Autodesk Inventor part; units mm, degrees
(part 2 of 3)
  line L717 (-49.225, -33.8) -> (-47.975, -33.8)
  line L718 (-47.975, -33.8) -> (-47.975, -32.7)
  line L719 (-47.975, -32.7) -> (-49.225, -32.7)
  arc A261 (-49.425, -32.5) -> (-49.225, -32.7) centre (-49.225, -32.5) ccw
  line L720 (-49.425, -32.5) -> (-49.425, -31.35)
  line L721 (-49.425, -31.35) -> (-50.325, -31.35)
  line L722 (-50.325, -31.35) -> (-50.325, -32.5)
  arc A262 (-50.525, -32.7) -> (-50.325, -32.5) centre (-50.525, -32.5) ccw
  line L723 (-50.525, -32.7) -> (-51.775, -32.7)
  line L724 (-51.775, -32.7) -> (-51.775, -33.8)
  line L725 (-51.775, -33.8) -> (-50.525, -33.8)
  arc A263 (-50.325, -34) -> (-50.525, -33.8) centre (-50.525, -34) ccw
  line L726 (-36.075, -53) -> (-36.075, -54.15)
  line L727 (-36.075, -54.15) -> (-35.175, -54.15)
  line L728 (-35.175, -54.15) -> (-35.175, -53)
  arc A264 (-34.975, -52.8) -> (-35.175, -53) centre (-34.975, -53) ccw
  line L729 (-34.975, -52.8) -> (-33.725, -52.8)
  line L730 (-33.725, -52.8) -> (-33.725, -51.7)
  line L731 (-33.725, -51.7) -> (-34.975, -51.7)
  arc A265 (-35.175, -51.5) -> (-34.975, -51.7) centre (-34.975, -51.5) ccw
  line L732 (-35.175, -51.5) -> (-35.175, -50.35)
  line L733 (-35.175, -50.35) -> (-36.075, -50.35)
  line L734 (-36.075, -50.35) -> (-36.075, -51.5)
  arc A266 (-36.275, -51.7) -> (-36.075, -51.5) centre (-36.275, -51.5) ccw
  line L735 (-36.275, -51.7) -> (-37.525, -51.7)
  line L736 (-37.525, -51.7) -> (-37.525, -52.8)
  line L737 (-37.525, -52.8) -> (-36.275, -52.8)
  arc A267 (-36.075, -53) -> (-36.275, -52.8) centre (-36.275, -53) ccw
  line L738 (-12.325, -53) -> (-12.325, -54.15)
  line L739 (-12.325, -54.15) -> (-11.425, -54.15)
  line L740 (-11.425, -54.15) -> (-11.425, -53)
  arc A268 (-11.225, -52.8) -> (-11.425, -53) centre (-11.225, -53) ccw
  line L741 (-11.225, -52.8) -> (-9.975, -52.8)
  line L742 (-9.975, -52.8) -> (-9.975, -51.7)
  line L743 (-9.975, -51.7) -> (-11.225, -51.7)
  arc A269 (-11.425, -51.5) -> (-11.225, -51.7) centre (-11.225, -51.5) ccw
  line L744 (-11.425, -51.5) -> (-11.425, -50.35)
  line L745 (-11.425, -50.35) -> (-12.325, -50.35)
  line L746 (-12.325, -50.35) -> (-12.325, -51.5)
  arc A270 (-12.525, -51.7) -> (-12.325, -51.5) centre (-12.525, -51.5) ccw
  line L747 (-12.525, -51.7) -> (-13.775, -51.7)
  line L748 (-13.775, -51.7) -> (-13.775, -52.8)
  line L749 (-13.775, -52.8) -> (-12.525, -52.8)
  arc A271 (-12.325, -53) -> (-12.525, -52.8) centre (-12.525, -53) ccw
  line L750 (-19.45, -34) -> (-19.45, -35.15)
  line L751 (-19.45, -35.15) -> (-18.55, -35.15)
  line L752 (-18.55, -35.15) -> (-18.55, -34)
  arc A272 (-18.35, -33.8) -> (-18.55, -34) centre (-18.35, -34) ccw
  line L753 (-18.35, -33.8) -> (-17.1, -33.8)
  line L754 (-17.1, -33.8) -> (-17.1, -32.7)
  line L755 (-17.1, -32.7) -> (-18.35, -32.7)
  arc A273 (-18.55, -32.5) -> (-18.35, -32.7) centre (-18.35, -32.5) ccw
  line L756 (-18.55, -32.5) -> (-18.55, -31.35)
  line L757 (-18.55, -31.35) -> (-19.45, -31.35)
  line L758 (-19.45, -31.35) -> (-19.45, -32.5)
  arc A274 (-19.65, -32.7) -> (-19.45, -32.5) centre (-19.65, -32.5) ccw
  line L759 (-19.65, -32.7) -> (-20.9, -32.7)
  line L760 (-20.9, -32.7) -> (-20.9, -33.8)
  line L761 (-20.9, -33.8) -> (-19.65, -33.8)
  arc A275 (-19.45, -34) -> (-19.65, -33.8) centre (-19.65, -34) ccw
  line L762 (-28.95, -15) -> (-28.95, -16.15)
  line L763 (-28.95, -16.15) -> (-28.05, -16.15)
  line L764 (-28.05, -16.15) -> (-28.05, -15)
  arc A276 (-27.85, -14.8) -> (-28.05, -15) centre (-27.85, -15) ccw
  line L765 (-27.85, -14.8) -> (-26.6, -14.8)
  line L766 (-26.6, -14.8) -> (-26.6, -13.7)
  line L767 (-26.6, -13.7) -> (-27.85, -13.7)
  arc A277 (-28.05, -13.5) -> (-27.85, -13.7) centre (-27.85, -13.5) ccw
  line L768 (-28.05, -13.5) -> (-28.05, -12.35)
  line L769 (-28.05, -12.35) -> (-28.95, -12.35)
  line L770 (-28.95, -12.35) -> (-28.95, -13.5)
  arc A278 (-29.15, -13.7) -> (-28.95, -13.5) centre (-29.15, -13.5) ccw
  line L771 (-29.15, -13.7) -> (-30.4, -13.7)
  line L772 (-30.4, -13.7) -> (-30.4, -14.8)
  line L773 (-30.4, -14.8) -> (-29.15, -14.8)
  arc A279 (-28.95, -15) -> (-29.15, -14.8) centre (-29.15, -15) ccw
  line L774 (-33.7, 4) -> (-33.7, 2.85)
  line L775 (-33.7, 2.85) -> (-32.8, 2.85)
  line L776 (-32.8, 2.85) -> (-32.8, 4)
  arc A280 (-32.6, 4.2) -> (-32.8, 4) centre (-32.6, 4) ccw
  line L777 (-32.6, 4.2) -> (-31.35, 4.2)
  line L778 (-31.35, 4.2) -> (-31.35, 5.3)
  line L779 (-31.35, 5.3) -> (-32.6, 5.3)
  arc A281 (-32.8, 5.5) -> (-32.6, 5.3) centre (-32.6, 5.5) ccw
  line L780 (-32.8, 5.5) -> (-32.8, 6.65)
  line L781 (-32.8, 6.65) -> (-33.7, 6.65)
  line L782 (-33.7, 6.65) -> (-33.7, 5.5)
  arc A282 (-33.9, 5.3) -> (-33.7, 5.5) centre (-33.9, 5.5) ccw
  line L783 (-33.9, 5.3) -> (-35.15, 5.3)
  line L784 (-35.15, 5.3) -> (-35.15, 4.2)
  line L785 (-35.15, 4.2) -> (-33.9, 4.2)
  arc A283 (-33.7, 4) -> (-33.9, 4.2) centre (-33.9, 4) ccw
  line L786 (-14.7, 4) -> (-14.7, 2.85)
  line L787 (-14.7, 2.85) -> (-13.8, 2.85)
  line L788 (-13.8, 2.85) -> (-13.8, 4)
  arc A284 (-13.6, 4.2) -> (-13.8, 4) centre (-13.6, 4) ccw
  line L789 (-13.6, 4.2) -> (-12.35, 4.2)
  line L790 (-12.35, 4.2) -> (-12.35, 5.3)
  line L791 (-12.35, 5.3) -> (-13.6, 5.3)
  arc A285 (-13.8, 5.5) -> (-13.6, 5.3) centre (-13.6, 5.5) ccw
  line L792 (-13.8, 5.5) -> (-13.8, 6.65)
  line L793 (-13.8, 6.65) -> (-14.7, 6.65)
  line L794 (-14.7, 6.65) -> (-14.7, 5.5)
  arc A286 (-14.9, 5.3) -> (-14.7, 5.5) centre (-14.9, 5.5) ccw
  line L795 (-14.9, 5.3) -> (-16.15, 5.3)
  line L796 (-16.15, 5.3) -> (-16.15, 4.2)
  line L797 (-16.15, 4.2) -> (-14.9, 4.2)
  arc A287 (-14.7, 4) -> (-14.9, 4.2) centre (-14.9, 4) ccw
  line L798 (-9.95, -15) -> (-9.95, -16.15)
  line L799 (-9.95, -16.15) -> (-9.05, -16.15)
  line L800 (-9.05, -16.15) -> (-9.05, -15)
  arc A288 (-8.85, -14.8) -> (-9.05, -15) centre (-8.85, -15) ccw
  line L801 (-8.85, -14.8) -> (-7.6, -14.8)
  line L802 (-7.6, -14.8) -> (-7.6, -13.7)
  line L803 (-7.6, -13.7) -> (-8.85, -13.7)
  arc A289 (-9.05, -13.5) -> (-8.85, -13.7) centre (-8.85, -13.5) ccw
  line L804 (-9.05, -13.5) -> (-9.05, -12.35)
  line L805 (-9.05, -12.35) -> (-9.95, -12.35)
  line L806 (-9.95, -12.35) -> (-9.95, -13.5)
  arc A290 (-10.15, -13.7) -> (-9.95, -13.5) centre (-10.15, -13.5) ccw
  line L807 (-10.15, -13.7) -> (-11.4, -13.7)
  line L808 (-11.4, -13.7) -> (-11.4, -14.8)
  line L809 (-11.4, -14.8) -> (-10.15, -14.8)
  arc A291 (-9.95, -15) -> (-10.15, -14.8) centre (-10.15, -15) ccw
  line L810 (9.05, -15) -> (9.05, -16.15)
  line L811 (9.05, -16.15) -> (9.95, -16.15)
  line L812 (9.95, -16.15) -> (9.95, -15)
  arc A292 (10.15, -14.8) -> (9.95, -15) centre (10.15, -15) ccw
  line L813 (10.15, -14.8) -> (11.4, -14.8)
  line L814 (11.4, -14.8) -> (11.4, -13.7)
  line L815 (11.4, -13.7) -> (10.15, -13.7)
  arc A293 (9.95, -13.5) -> (10.15, -13.7) centre (10.15, -13.5) ccw
  line L816 (9.95, -13.5) -> (9.95, -12.35)
  line L817 (9.95, -12.35) -> (9.05, -12.35)
  line L818 (9.05, -12.35) -> (9.05, -13.5)
  arc A294 (8.85, -13.7) -> (9.05, -13.5) centre (8.85, -13.5) ccw
  line L819 (8.85, -13.7) -> (7.6, -13.7)
  line L820 (7.6, -13.7) -> (7.6, -14.8)
  line L821 (7.6, -14.8) -> (8.85, -14.8)
  arc A295 (9.05, -15) -> (8.85, -14.8) centre (8.85, -15) ccw
  line L822 (4.3, 4) -> (4.3, 2.85)
  line L823 (4.3, 2.85) -> (5.2, 2.85)
  line L824 (5.2, 2.85) -> (5.2, 4)
  arc A296 (5.4, 4.2) -> (5.2, 4) centre (5.4, 4) ccw
  line L825 (5.4, 4.2) -> (6.65, 4.2)
  line L826 (6.65, 4.2) -> (6.65, 5.3)
  line L827 (6.65, 5.3) -> (5.4, 5.3)
  arc A297 (5.2, 5.5) -> (5.4, 5.3) centre (5.4, 5.5) ccw
  line L828 (5.2, 5.5) -> (5.2, 6.65)
  line L829 (5.2, 6.65) -> (4.3, 6.65)
  line L830 (4.3, 6.65) -> (4.3, 5.5)
  arc A298 (4.1, 5.3) -> (4.3, 5.5) centre (4.1, 5.5) ccw
  line L831 (4.1, 5.3) -> (2.85, 5.3)
  line L832 (2.85, 5.3) -> (2.85, 4.2)
  line L833 (2.85, 4.2) -> (4.1, 4.2)
  arc A299 (4.3, 4) -> (4.1, 4.2) centre (4.1, 4) ccw
  line L834 (-0.45, -34) -> (-0.45, -35.15)
  line L835 (-0.45, -35.15) -> (0.45, -35.15)
  line L836 (0.45, -35.15) -> (0.45, -34)
  arc A300 (0.65, -33.8) -> (0.45, -34) centre (0.65, -34) ccw
  line L837 (0.65, -33.8) -> (1.9, -33.8)
  line L838 (1.9, -33.8) -> (1.9, -32.7)
  line L839 (1.9, -32.7) -> (0.65, -32.7)
  arc A301 (0.45, -32.5) -> (0.65, -32.7) centre (0.65, -32.5) ccw
  line L840 (0.45, -32.5) -> (0.45, -31.35)
  line L841 (0.45, -31.35) -> (-0.45, -31.35)
  line L842 (-0.45, -31.35) -> (-0.45, -32.5)
  arc A302 (-0.65, -32.7) -> (-0.45, -32.5) centre (-0.65, -32.5) ccw
  line L843 (-0.65, -32.7) -> (-1.9, -32.7)
  line L844 (-1.9, -32.7) -> (-1.9, -33.8)
  line L845 (-1.9, -33.8) -> (-0.65, -33.8)
  arc A303 (-0.45, -34) -> (-0.65, -33.8) centre (-0.65, -34) ccw
  line L846 (18.55, -34) -> (18.55, -35.15)
  line L847 (18.55, -35.15) -> (19.45, -35.15)
  line L848 (19.45, -35.15) -> (19.45, -34)
  arc A304 (19.65, -33.8) -> (19.45, -34) centre (19.65, -34) ccw
  line L849 (19.65, -33.8) -> (20.9, -33.8)
  line L850 (20.9, -33.8) -> (20.9, -32.7)
  line L851 (20.9, -32.7) -> (19.65, -32.7)
  arc A305 (19.45, -32.5) -> (19.65, -32.7) centre (19.65, -32.5) ccw
  line L852 (19.45, -32.5) -> (19.45, -31.35)
  line L853 (19.45, -31.35) -> (18.55, -31.35)
  line L854 (18.55, -31.35) -> (18.55, -32.5)
  arc A306 (18.35, -32.7) -> (18.55, -32.5) centre (18.35, -32.5) ccw
  line L855 (18.35, -32.7) -> (17.1, -32.7)
  line L856 (17.1, -32.7) -> (17.1, -33.8)
  line L857 (17.1, -33.8) -> (18.35, -33.8)
  arc A307 (18.55, -34) -> (18.35, -33.8) centre (18.35, -34) ccw
  line L858 (28.05, -15) -> (28.05, -16.15)
  line L859 (28.05, -16.15) -> (28.95, -16.15)
  line L860 (28.95, -16.15) -> (28.95, -15)
  arc A308 (29.15, -14.8) -> (28.95, -15) centre (29.15, -15) ccw
  line L861 (29.15, -14.8) -> (30.4, -14.8)
  line L862 (30.4, -14.8) -> (30.4, -13.7)
  line L863 (30.4, -13.7) -> (29.15, -13.7)
  arc A309 (28.95, -13.5) -> (29.15, -13.7) centre (29.15, -13.5) ccw
  line L864 (28.95, -13.5) -> (28.95, -12.35)
  line L865 (28.95, -12.35) -> (28.05, -12.35)
  line L866 (28.05, -12.35) -> (28.05, -13.5)
  arc A310 (27.85, -13.7) -> (28.05, -13.5) centre (27.85, -13.5) ccw
  line L867 (27.85, -13.7) -> (26.6, -13.7)
  line L868 (26.6, -13.7) -> (26.6, -14.8)
  line L869 (26.6, -14.8) -> (27.85, -14.8)
  arc A311 (28.05, -15) -> (27.85, -14.8) centre (27.85, -15) ccw
  line L870 (23.3, 4) -> (23.3, 2.85)
  line L871 (23.3, 2.85) -> (24.2, 2.85)
  line L872 (24.2, 2.85) -> (24.2, 4)
  arc A312 (24.4, 4.2) -> (24.2, 4) centre (24.4, 4) ccw
  line L873 (24.4, 4.2) -> (25.65, 4.2)
  line L874 (25.65, 4.2) -> (25.65, 5.3)
  line L875 (25.65, 5.3) -> (24.4, 5.3)
  arc A313 (24.2, 5.5) -> (24.4, 5.3) centre (24.4, 5.5) ccw
  line L876 (24.2, 5.5) -> (24.2, 6.65)
  line L877 (24.2, 6.65) -> (23.3, 6.65)
  line L878 (23.3, 6.65) -> (23.3, 5.5)
  arc A314 (23.1, 5.3) -> (23.3, 5.5) centre (23.1, 5.5) ccw
  line L879 (23.1, 5.3) -> (21.85, 5.3)
  line L880 (21.85, 5.3) -> (21.85, 4.2)
  line L881 (21.85, 4.2) -> (23.1, 4.2)
  arc A315 (23.3, 4) -> (23.1, 4.2) centre (23.1, 4) ccw
  line L882 (37.55, -34) -> (37.55, -35.15)
  line L883 (37.55, -35.15) -> (38.45, -35.15)
  line L884 (38.45, -35.15) -> (38.45, -34)
  arc A316 (38.65, -33.8) -> (38.45, -34) centre (38.65, -34) ccw
  line L885 (38.65, -33.8) -> (39.9, -33.8)
  line L886 (39.9, -33.8) -> (39.9, -32.7)
  line L887 (39.9, -32.7) -> (38.65, -32.7)
  arc A317 (38.45, -32.5) -> (38.65, -32.7) centre (38.65, -32.5) ccw
  line L888 (38.45, -32.5) -> (38.45, -31.35)
  line L889 (38.45, -31.35) -> (37.55, -31.35)
  line L890 (37.55, -31.35) -> (37.55, -32.5)
  arc A318 (37.35, -32.7) -> (37.55, -32.5) centre (37.35, -32.5) ccw
  line L891 (37.35, -32.7) -> (36.1, -32.7)
  line L892 (36.1, -32.7) -> (36.1, -33.8)
  line L893 (36.1, -33.8) -> (37.35, -33.8)
  arc A319 (37.55, -34) -> (37.35, -33.8) centre (37.35, -34) ccw
  line L894 (47.05, -15) -> (47.05, -16.15)
  line L895 (47.05, -16.15) -> (47.95, -16.15)
  line L896 (47.95, -16.15) -> (47.95, -15)
  arc A320 (48.15, -14.8) -> (47.95, -15) centre (48.15, -15) ccw
  line L897 (48.15, -14.8) -> (49.4, -14.8)
  line L898 (49.4, -14.8) -> (49.4, -13.7)
  line L899 (49.4, -13.7) -> (48.15, -13.7)
  arc A321 (47.95, -13.5) -> (48.15, -13.7) centre (48.15, -13.5) ccw
  line L900 (47.95, -13.5) -> (47.95, -12.35)
  line L901 (47.95, -12.35) -> (47.05, -12.35)
  line L902 (47.05, -12.35) -> (47.05, -13.5)
  arc A322 (46.85, -13.7) -> (47.05, -13.5) centre (46.85, -13.5) ccw
  line L903 (46.85, -13.7) -> (45.6, -13.7)
  line L904 (45.6, -13.7) -> (45.6, -14.8)
  line L905 (45.6, -14.8) -> (46.85, -14.8)
  arc A323 (47.05, -15) -> (46.85, -14.8) centre (46.85, -15) ccw
  line L906 (42.3, 4) -> (42.3, 2.85)
  line L907 (42.3, 2.85) -> (43.2, 2.85)
  line L908 (43.2, 2.85) -> (43.2, 4)
  arc A324 (43.4, 4.2) -> (43.2, 4) centre (43.4, 4) ccw
  line L909 (43.4, 4.2) -> (44.65, 4.2)
  line L910 (44.65, 4.2) -> (44.65, 5.3)
  line L911 (44.65, 5.3) -> (43.4, 5.3)
  arc A325 (43.2, 5.5) -> (43.4, 5.3) centre (43.4, 5.5) ccw
  line L912 (43.2, 5.5) -> (43.2, 6.65)
  line L913 (43.2, 6.65) -> (42.3, 6.65)
  line L914 (42.3, 6.65) -> (42.3, 5.5)
  arc A326 (42.1, 5.3) -> (42.3, 5.5) centre (42.1, 5.5) ccw
  line L915 (42.1, 5.3) -> (40.85, 5.3)
  line L916 (40.85, 5.3) -> (40.85, 4.2)
  line L917 (40.85, 4.2) -> (42.1, 4.2)
  arc A327 (42.3, 4) -> (42.1, 4.2) centre (42.1, 4) ccw
  line L918 (61.3, 4) -> (61.3, 2.85)
  line L919 (61.3, 2.85) -> (62.2, 2.85)
  line L920 (62.2, 2.85) -> (62.2, 4)
  arc A328 (62.4, 4.2) -> (62.2, 4) centre (62.4, 4) ccw
  line L921 (62.4, 4.2) -> (63.65, 4.2)
  line L922 (63.65, 4.2) -> (63.65, 5.3)
  line L923 (63.65, 5.3) -> (62.4, 5.3)
  arc A329 (62.2, 5.5) -> (62.4, 5.3) centre (62.4, 5.5) ccw
  line L924 (62.2, 5.5) -> (62.2, 6.65)
  line L925 (62.2, 6.65) -> (61.3, 6.65)
  line L926 (61.3, 6.65) -> (61.3, 5.5)
  arc A330 (61.1, 5.3) -> (61.3, 5.5) centre (61.1, 5.5) ccw
  line L927 (61.1, 5.3) -> (59.85, 5.3)
  line L928 (59.85, 5.3) -> (59.85, 4.2)
  line L929 (59.85, 4.2) -> (61.1, 4.2)
  arc A331 (61.3, 4) -> (61.1, 4.2) centre (61.1, 4) ccw
  line L930 (80.3, 4) -> (80.3, 2.85)
  line L931 (80.3, 2.85) -> (81.2, 2.85)
  line L932 (81.2, 2.85) -> (81.2, 4)
  arc A332 (81.4, 4.2) -> (81.2, 4) centre (81.4, 4) ccw
  line L933 (81.4, 4.2) -> (82.65, 4.2)
  line L934 (82.65, 4.2) -> (82.65, 5.3)
  line L935 (82.65, 5.3) -> (81.4, 5.3)
  arc A333 (81.2, 5.5) -> (81.4, 5.3) centre (81.4, 5.5) ccw
  line L936 (81.2, 5.5) -> (81.2, 6.65)
  line L937 (81.2, 6.65) -> (80.3, 6.65)
  line L938 (80.3, 6.65) -> (80.3, 5.5)
  arc A334 (80.1, 5.3) -> (80.3, 5.5) centre (80.1, 5.5) ccw
  line L939 (80.1, 5.3) -> (78.85, 5.3)
  line L940 (78.85, 5.3) -> (78.85, 4.2)
  line L941 (78.85, 4.2) -> (80.1, 4.2)
  arc A335 (80.3, 4) -> (80.1, 4.2) centre (80.1, 4) ccw
  line L942 (85.05, -15) -> (85.05, -16.15)
  line L943 (85.05, -16.15) -> (85.95, -16.15)
  line L944 (85.95, -16.15) -> (85.95, -15)
  arc A336 (86.15, -14.8) -> (85.95, -15) centre (86.15, -15) ccw
  line L945 (86.15, -14.8) -> (87.4, -14.8)
  line L946 (87.4, -14.8) -> (87.4, -13.7)
  line L947 (87.4, -13.7) -> (86.15, -13.7)
  arc A337 (85.95, -13.5) -> (86.15, -13.7) centre (86.15, -13.5) ccw
  line L948 (85.95, -13.5) -> (85.95, -12.35)
  line L949 (85.95, -12.35) -> (85.05, -12.35)
  line L950 (85.05, -12.35) -> (85.05, -13.5)
  arc A338 (84.85, -13.7) -> (85.05, -13.5) centre (84.85, -13.5) ccw
  line L951 (84.85, -13.7) -> (83.6, -13.7)
  line L952 (83.6, -13.7) -> (83.6, -14.8)
  line L953 (83.6, -14.8) -> (84.85, -14.8)
  arc A339 (85.05, -15) -> (84.85, -14.8) centre (84.85, -15) ccw
  line L954 (66.05, -15) -> (66.05, -16.15)
  line L955 (66.05, -16.15) -> (66.95, -16.15)
  line L956 (66.95, -16.15) -> (66.95, -15)
  arc A340 (67.15, -14.8) -> (66.95, -15) centre (67.15, -15) ccw
  line L957 (67.15, -14.8) -> (68.4, -14.8)
  line L958 (68.4, -14.8) -> (68.4, -13.7)
  line L959 (68.4, -13.7) -> (67.15, -13.7)
  arc A341 (66.95, -13.5) -> (67.15, -13.7) centre (67.15, -13.5) ccw
  line L960 (66.95, -13.5) -> (66.95, -12.35)
  line L961 (66.95, -12.35) -> (66.05, -12.35)
  line L962 (66.05, -12.35) -> (66.05, -13.5)
  arc A342 (65.85, -13.7) -> (66.05, -13.5) centre (65.85, -13.5) ccw
  line L963 (65.85, -13.7) -> (64.6, -13.7)
  line L964 (64.6, -13.7) -> (64.6, -14.8)
  line L965 (64.6, -14.8) -> (65.85, -14.8)
  arc A343 (66.05, -15) -> (65.85, -14.8) centre (65.85, -15) ccw
  line L966 (56.55, -34) -> (56.55, -35.15)
  line L967 (56.55, -35.15) -> (57.45, -35.15)
  line L968 (57.45, -35.15) -> (57.45, -34)
  arc A344 (57.65, -33.8) -> (57.45, -34) centre (57.65, -34) ccw
  line L969 (57.65, -33.8) -> (58.9, -33.8)
  line L970 (58.9, -33.8) -> (58.9, -32.7)
  line L971 (58.9, -32.7) -> (57.65, -32.7)
  arc A345 (57.45, -32.5) -> (57.65, -32.7) centre (57.65, -32.5) ccw
  line L972 (57.45, -32.5) -> (57.45, -31.35)
  line L973 (57.45, -31.35) -> (56.55, -31.35)
  line L974 (56.55, -31.35) -> (56.55, -32.5)
  arc A346 (56.35, -32.7) -> (56.55, -32.5) centre (56.35, -32.5) ccw
  line L975 (56.35, -32.7) -> (55.1, -32.7)
  line L976 (55.1, -32.7) -> (55.1, -33.8)
  line L977 (55.1, -33.8) -> (56.35, -33.8)
  arc A347 (56.55, -34) -> (56.35, -33.8) centre (56.35, -34) ccw
  line L978 (75.55, -34) -> (75.55, -35.15)
  line L979 (75.55, -35.15) -> (76.45, -35.15)
  line L980 (76.45, -35.15) -> (76.45, -34)
  arc A348 (76.65, -33.8) -> (76.45, -34) centre (76.65, -34) ccw
  line L981 (76.65, -33.8) -> (77.9, -33.8)
  line L982 (77.9, -33.8) -> (77.9, -32.7)
  line L983 (77.9, -32.7) -> (76.65, -32.7)
  arc A349 (76.45, -32.5) -> (76.65, -32.7) centre (76.65, -32.5) ccw
  line L984 (76.45, -32.5) -> (76.45, -31.35)
  line L985 (76.45, -31.35) -> (75.55, -31.35)
  line L986 (75.55, -31.35) -> (75.55, -32.5)
  arc A350 (75.35, -32.7) -> (75.55, -32.5) centre (75.35, -32.5) ccw
  line L987 (75.35, -32.7) -> (74.1, -32.7)
  line L988 (74.1, -32.7) -> (74.1, -33.8)
  line L989 (74.1, -33.8) -> (75.35, -33.8)
  arc A351 (75.55, -34) -> (75.35, -33.8) centre (75.35, -34) ccw
  line L990 (94.55, -34) -> (94.55, -35.15)
  line L991 (94.55, -35.15) -> (95.45, -35.15)
  line L992 (95.45, -35.15) -> (95.45, -34)
  arc A352 (95.65, -33.8) -> (95.45, -34) centre (95.65, -34) ccw
  line L993 (95.65, -33.8) -> (96.9, -33.8)
  line L994 (96.9, -33.8) -> (96.9, -32.7)
  line L995 (96.9, -32.7) -> (95.65, -32.7)
  arc A353 (95.45, -32.5) -> (95.65, -32.7) centre (95.65, -32.5) ccw
  line L996 (95.45, -32.5) -> (95.45, -31.35)
  line L997 (95.45, -31.35) -> (94.55, -31.35)
  line L998 (94.55, -31.35) -> (94.55, -32.5)
  arc A354 (94.35, -32.7) -> (94.55, -32.5) centre (94.35, -32.5) ccw
  line L999 (94.35, -32.7) -> (93.1, -32.7)
  line L1000 (93.1, -32.7) -> (93.1, -33.8)
  line L1001 (93.1, -33.8) -> (94.35, -33.8)
  arc A355 (94.55, -34) -> (94.35, -33.8) centre (94.35, -34) ccw
  line L1002 (104.05, -15) -> (104.05, -16.15)
  line L1003 (104.05, -16.15) -> (104.95, -16.15)
  line L1004 (104.95, -16.15) -> (104.95, -15)
  arc A356 (105.15, -14.8) -> (104.95, -15) centre (105.15, -15) ccw
  line L1005 (105.15, -14.8) -> (106.4, -14.8)
  line L1006 (106.4, -14.8) -> (106.4, -13.7)
  line L1007 (106.4, -13.7) -> (105.15, -13.7)
  arc A357 (104.95, -13.5) -> (105.15, -13.7) centre (105.15, -13.5) ccw
  line L1008 (104.95, -13.5) -> (104.95, -12.35)
  line L1009 (104.95, -12.35) -> (104.05, -12.35)
  line L1010 (104.05, -12.35) -> (104.05, -13.5)
  arc A358 (103.85, -13.7) -> (104.05, -13.5) centre (103.85, -13.5) ccw
  line L1011 (103.85, -13.7) -> (102.6, -13.7)
  line L1012 (102.6, -13.7) -> (102.6, -14.8)
  line L1013 (102.6, -14.8) -> (103.85, -14.8)
  arc A359 (104.05, -15) -> (103.85, -14.8) centre (103.85, -15) ccw
  line L1014 (99.3, 4) -> (99.3, 2.85)
  line L1015 (99.3, 2.85) -> (100.2, 2.85)
  line L1016 (100.2, 2.85) -> (100.2, 4)
  arc A360 (100.4, 4.2) -> (100.2, 4) centre (100.4, 4) ccw
  line L1017 (100.4, 4.2) -> (101.65, 4.2)
  line L1018 (101.65, 4.2) -> (101.65, 5.3)
  line L1019 (101.65, 5.3) -> (100.4, 5.3)
  arc A361 (100.2, 5.5) -> (100.4, 5.3) centre (100.4, 5.5) ccw
  line L1020 (100.2, 5.5) -> (100.2, 6.65)
  line L1021 (100.2, 6.65) -> (99.3, 6.65)
  line L1022 (99.3, 6.65) -> (99.3, 5.5)
  arc A362 (99.1, 5.3) -> (99.3, 5.5) centre (99.1, 5.5) ccw
  line L1023 (99.1, 5.3) -> (97.85, 5.3)
  line L1024 (97.85, 5.3) -> (97.85, 4.2)
  line L1025 (97.85, 4.2) -> (99.1, 4.2)
  arc A363 (99.3, 4) -> (99.1, 4.2) centre (99.1, 4) ccw
  line L1026 (118.3, 4) -> (118.3, 2.85)
  line L1027 (118.3, 2.85) -> (119.2, 2.85)
  line L1028 (119.2, 2.85) -> (119.2, 4)
  arc A364 (119.4, 4.2) -> (119.2, 4) centre (119.4, 4) ccw
  line L1029 (119.4, 4.2) -> (120.65, 4.2)
  line L1030 (120.65, 4.2) -> (120.65, 5.3)
  line L1031 (120.65, 5.3) -> (119.4, 5.3)
  arc A365 (119.2, 5.5) -> (119.4, 5.3) centre (119.4, 5.5) ccw
  line L1032 (119.2, 5.5) -> (119.2, 6.65)
  line L1033 (119.2, 6.65) -> (118.3, 6.65)
  line L1034 (118.3, 6.65) -> (118.3, 5.5)
  arc A366 (118.1, 5.3) -> (118.3, 5.5) centre (118.1, 5.5) ccw
  line L1035 (118.1, 5.3) -> (116.85, 5.3)
  line L1036 (116.85, 5.3) -> (116.85, 4.2)
  line L1037 (116.85, 4.2) -> (118.1, 4.2)
  arc A367 (118.3, 4) -> (118.1, 4.2) centre (118.1, 4) ccw
  line L1038 (137.3, 4) -> (137.3, 2.85)
  line L1039 (137.3, 2.85) -> (138.2, 2.85)
  line L1040 (138.2, 2.85) -> (138.2, 4)
  arc A368 (138.4, 4.2) -> (138.2, 4) centre (138.4, 4) ccw
  line L1041 (138.4, 4.2) -> (139.65, 4.2)
  line L1042 (139.65, 4.2) -> (139.65, 5.3)
  line L1043 (139.65, 5.3) -> (138.4, 5.3)
  arc A369 (138.2, 5.5) -> (138.4, 5.3) centre (138.4, 5.5) ccw
  line L1044 (138.2, 5.5) -> (138.2, 6.65)
  line L1045 (138.2, 6.65) -> (137.3, 6.65)
  line L1046 (137.3, 6.65) -> (137.3, 5.5)
  arc A370 (137.1, 5.3) -> (137.3, 5.5) centre (137.1, 5.5) ccw
  line L1047 (137.1, 5.3) -> (135.85, 5.3)
  line L1048 (135.85, 5.3) -> (135.85, 4.2)
  line L1049 (135.85, 4.2) -> (137.1, 4.2)
  arc A371 (137.3, 4) -> (137.1, 4.2) centre (137.1, 4) ccw
  line L1050 (123.05, -15) -> (123.05, -16.15)
  line L1051 (123.05, -16.15) -> (123.95, -16.15)
  line L1052 (123.95, -16.15) -> (123.95, -15)
  arc A372 (124.15, -14.8) -> (123.95, -15) centre (124.15, -15) ccw
  line L1053 (124.15, -14.8) -> (125.4, -14.8)
  line L1054 (125.4, -14.8) -> (125.4, -13.7)
  line L1055 (125.4, -13.7) -> (124.15, -13.7)
  arc A373 (123.95, -13.5) -> (124.15, -13.7) centre (124.15, -13.5) ccw
  line L1056 (123.95, -13.5) -> (123.95, -12.35)
  line L1057 (123.95, -12.35) -> (123.05, -12.35)
  line L1058 (123.05, -12.35) -> (123.05, -13.5)
  arc A374 (122.85, -13.7) -> (123.05, -13.5) centre (122.85, -13.5) ccw
  line L1059 (122.85, -13.7) -> (121.6, -13.7)
  line L1060 (121.6, -13.7) -> (121.6, -14.8)
  line L1061 (121.6, -14.8) -> (122.85, -14.8)
  arc A375 (123.05, -15) -> (122.85, -14.8) centre (122.85, -15) ccw
  line L1062 (142.05, -15) -> (142.05, -16.15)
  line L1063 (142.05, -16.15) -> (142.95, -16.15)
  line L1064 (142.95, -16.15) -> (142.95, -15)
  arc A376 (143.15, -14.8) -> (142.95, -15) centre (143.15, -15) ccw
  line L1065 (143.15, -14.8) -> (144.4, -14.8)
  line L1066 (144.4, -14.8) -> (144.4, -13.7)
  line L1067 (144.4, -13.7) -> (143.15, -13.7)
  arc A377 (142.95, -13.5) -> (143.15, -13.7) centre (143.15, -13.5) ccw
  line L1068 (142.95, -13.5) -> (142.95, -12.35)
  line L1069 (142.95, -12.35) -> (142.05, -12.35)
  line L1070 (142.05, -12.35) -> (142.05, -13.5)
  arc A378 (141.85, -13.7) -> (142.05, -13.5) centre (141.85, -13.5) ccw
  line L1071 (141.85, -13.7) -> (140.6, -13.7)
  line L1072 (140.6, -13.7) -> (140.6, -14.8)
  line L1073 (140.6, -14.8) -> (141.85, -14.8)
  arc A379 (142.05, -15) -> (141.85, -14.8) centre (141.85, -15) ccw
  line L1074 (156.3, 4) -> (156.3, 2.85)
  line L1075 (156.3, 2.85) -> (157.2, 2.85)
  line L1076 (157.2, 2.85) -> (157.2, 4)
  arc A380 (157.4, 4.2) -> (157.2, 4) centre (157.4, 4) ccw
  line L1077 (157.4, 4.2) -> (158.65, 4.2)
  line L1078 (158.65, 4.2) -> (158.65, 5.3)
  line L1079 (158.65, 5.3) -> (157.4, 5.3)
  arc A381 (157.2, 5.5) -> (157.4, 5.3) centre (157.4, 5.5) ccw
  line L1080 (157.2, 5.5) -> (157.2, 6.65)
  line L1081 (157.2, 6.65) -> (156.3, 6.65)
  line L1082 (156.3, 6.65) -> (156.3, 5.5)
  arc A382 (156.1, 5.3) -> (156.3, 5.5) centre (156.1, 5.5) ccw
  line L1083 (156.1, 5.3) -> (154.85, 5.3)
  line L1084 (154.85, 5.3) -> (154.85, 4.2)
  line L1085 (154.85, 4.2) -> (156.1, 4.2)
  arc A383 (156.3, 4) -> (156.1, 4.2) centre (156.1, 4) ccw
  line L1086 (161.05, -15) -> (161.05, -16.15)
  line L1087 (161.05, -16.15) -> (161.95, -16.15)
  line L1088 (161.95, -16.15) -> (161.95, -15)
  arc A384 (162.15, -14.8) -> (161.95, -15) centre (162.15, -15) ccw
  line L1089 (162.15, -14.8) -> (163.4, -14.8)
  line L1090 (163.4, -14.8) -> (163.4, -13.7)
  line L1091 (163.4, -13.7) -> (162.15, -13.7)
  arc A385 (161.95, -13.5) -> (162.15, -13.7) centre (162.15, -13.5) ccw
  line L1092 (161.95, -13.5) -> (161.95, -12.35)
  line L1093 (161.95, -12.35) -> (161.05, -12.35)
  line L1094 (161.05, -12.35) -> (161.05, -13.5)
  arc A386 (160.85, -13.7) -> (161.05, -13.5) centre (160.85, -13.5) ccw
  line L1095 (160.85, -13.7) -> (159.6, -13.7)
  line L1096 (159.6, -13.7) -> (159.6, -14.8)
  line L1097 (159.6, -14.8) -> (160.85, -14.8)
  arc A387 (161.05, -15) -> (160.85, -14.8) centre (160.85, -15) ccw
  line L1098 (113.55, -34) -> (113.55, -35.15)
  line L1099 (113.55, -35.15) -> (114.45, -35.15)
  line L1100 (114.45, -35.15) -> (114.45, -34)
  arc A388 (114.65, -33.8) -> (114.45, -34) centre (114.65, -34) ccw
  line L1101 (114.65, -33.8) -> (115.9, -33.8)
  line L1102 (115.9, -33.8) -> (115.9, -32.7)
  line L1103 (115.9, -32.7) -> (114.65, -32.7)
  arc A389 (114.45, -32.5) -> (114.65, -32.7) centre (114.65, -32.5) ccw
  line L1104 (114.45, -32.5) -> (114.45, -31.35)
  line L1105 (114.45, -31.35) -> (113.55, -31.35)
  line L1106 (113.55, -31.35) -> (113.55, -32.5)
  arc A390 (113.35, -32.7) -> (113.55, -32.5) centre (113.35, -32.5) ccw
  line L1107 (113.35, -32.7) -> (112.1, -32.7)
  line L1108 (112.1, -32.7) -> (112.1, -33.8)
  line L1109 (112.1, -33.8) -> (113.35, -33.8)
  arc A391 (113.55, -34) -> (113.35, -33.8) centre (113.35, -34) ccw
  line L1110 (132.55, -34) -> (132.55, -35.15)
  line L1111 (132.55, -35.15) -> (133.45, -35.15)
  line L1112 (133.45, -35.15) -> (133.45, -34)
  arc A392 (133.65, -33.8) -> (133.45, -34) centre (133.65, -34) ccw
  line L1113 (133.65, -33.8) -> (134.9, -33.8)
  line L1114 (134.9, -33.8) -> (134.9, -32.7)
  line L1115 (134.9, -32.7) -> (133.65, -32.7)
  arc A393 (133.45, -32.5) -> (133.65, -32.7) centre (133.65, -32.5) ccw
  line L1116 (133.45, -32.5) -> (133.45, -31.35)
  line L1117 (133.45, -31.35) -> (132.55, -31.35)
  line L1118 (132.55, -31.35) -> (132.55, -32.5)
  arc A394 (132.35, -32.7) -> (132.55, -32.5) centre (132.35, -32.5) ccw
  line L1119 (132.35, -32.7) -> (131.1, -32.7)
  line L1120 (131.1, -32.7) -> (131.1, -33.8)
  line L1121 (131.1, -33.8) -> (132.35, -33.8)
  arc A395 (132.55, -34) -> (132.35, -33.8) centre (132.35, -34) ccw
  line L1122 (151.55, -34) -> (151.55, -35.15)
  line L1123 (151.55, -35.15) -> (152.45, -35.15)
  line L1124 (152.45, -35.15) -> (152.45, -34)
  arc A396 (152.65, -33.8) -> (152.45, -34) centre (152.65, -34) ccw
  line L1125 (152.65, -33.8) -> (153.9, -33.8)
  line L1126 (153.9, -33.8) -> (153.9, -32.7)
  line L1127 (153.9, -32.7) -> (152.65, -32.7)
  arc A397 (152.45, -32.5) -> (152.65, -32.7) centre (152.65, -32.5) ccw
  line L1128 (152.45, -32.5) -> (152.45, -31.35)
  line L1129 (152.45, -31.35) -> (151.55, -31.35)
  line L1130 (151.55, -31.35) -> (151.55, -32.5)
  arc A398 (151.35, -32.7) -> (151.55, -32.5) centre (151.35, -32.5) ccw
  line L1131 (151.35, -32.7) -> (150.1, -32.7)
  line L1132 (150.1, -32.7) -> (150.1, -33.8)
  line L1133 (150.1, -33.8) -> (151.35, -33.8)
  arc A399 (151.55, -34) -> (151.35, -33.8) centre (151.35, -34) ccw
  line L1134 (175.3, 4) -> (175.3, 2.85)
  line L1135 (175.3, 2.85) -> (176.2, 2.85)
  line L1136 (176.2, 2.85) -> (176.2, 4)
  arc A400 (176.4, 4.2) -> (176.2, 4) centre (176.4, 4) ccw
  line L1137 (176.4, 4.2) -> (177.65, 4.2)
  line L1138 (177.65, 4.2) -> (177.65, 5.3)
  line L1139 (177.65, 5.3) -> (176.4, 5.3)
  arc A401 (176.2, 5.5) -> (176.4, 5.3) centre (176.4, 5.5) ccw
  line L1140 (176.2, 5.5) -> (176.2, 6.65)
  line L1141 (176.2, 6.65) -> (175.3, 6.65)
  line L1142 (175.3, 6.65) -> (175.3, 5.5)
  arc A402 (175.1, 5.3) -> (175.3, 5.5) centre (175.1, 5.5) ccw
  line L1143 (175.1, 5.3) -> (173.85, 5.3)
  line L1144 (173.85, 5.3) -> (173.85, 4.2)
  line L1145 (173.85, 4.2) -> (175.1, 4.2)
  arc A403 (175.3, 4) -> (175.1, 4.2) centre (175.1, 4) ccw
  line L1146 (199.05, 4) -> (199.05, 2.85)
  line L1147 (199.05, 2.85) -> (199.95, 2.85)
  line L1148 (199.95, 2.85) -> (199.95, 4)
  arc A404 (200.15, 4.2) -> (199.95, 4) centre (200.15, 4) ccw
  line L1149 (200.15, 4.2) -> (201.4, 4.2)
  line L1150 (201.4, 4.2) -> (201.4, 5.3)
  line L1151 (201.4, 5.3) -> (200.15, 5.3)
  arc A405 (199.95, 5.5) -> (200.15, 5.3) centre (200.15, 5.5) ccw
  line L1152 (199.95, 5.5) -> (199.95, 6.65)
  line L1153 (199.95, 6.65) -> (199.05, 6.65)
  line L1154 (199.05, 6.65) -> (199.05, 5.5)
  arc A406 (198.85, 5.3) -> (199.05, 5.5) centre (198.85, 5.5) ccw
  line L1155 (198.85, 5.3) -> (197.6, 5.3)
  line L1156 (197.6, 5.3) -> (197.6, 4.2)
  line L1157 (197.6, 4.2) -> (198.85, 4.2)
  arc A407 (199.05, 4) -> (198.85, 4.2) centre (198.85, 4) ccw
  line L1158 (191.925, -15) -> (191.925, -16.15)
  line L1159 (191.925, -16.15) -> (192.825, -16.15)
  line L1160 (192.825, -16.15) -> (192.825, -15)
  arc A408 (193.025, -14.8) -> (192.825, -15) centre (193.025, -15) ccw
  line L1161 (193.025, -14.8) -> (194.275, -14.8)
  line L1162 (194.275, -14.8) -> (194.275, -13.7)
  line L1163 (194.275, -13.7) -> (193.025, -13.7)
  arc A409 (192.825, -13.5) -> (193.025, -13.7) centre (193.025, -13.5) ccw
  line L1164 (192.825, -13.5) -> (192.825, -12.35)
  line L1165 (192.825, -12.35) -> (191.925, -12.35)
  line L1166 (191.925, -12.35) -> (191.925, -13.5)
  arc A410 (191.725, -13.7) -> (191.925, -13.5) centre (191.725, -13.5) ccw
  line L1167 (191.725, -13.7) -> (190.475, -13.7)
  line L1168 (190.475, -13.7) -> (190.475, -14.8)
  line L1169 (190.475, -14.8) -> (191.725, -14.8)
  arc A411 (191.925, -15) -> (191.725, -14.8) centre (191.725, -15) ccw
  line L1170 (187.175, -34) -> (187.175, -35.15)
  line L1171 (187.175, -35.15) -> (188.075, -35.15)
  line L1172 (188.075, -35.15) -> (188.075, -34)
  arc A412 (188.275, -33.8) -> (188.075, -34) centre (188.275, -34) ccw
  line L1173 (188.275, -33.8) -> (189.525, -33.8)
  line L1174 (189.525, -33.8) -> (189.525, -32.7)
  line L1175 (189.525, -32.7) -> (188.275, -32.7)
  arc A413 (188.075, -32.5) -> (188.275, -32.7) centre (188.275, -32.5) ccw
  line L1176 (188.075, -32.5) -> (188.075, -31.35)
  line L1177 (188.075, -31.35) -> (187.175, -31.35)
  line L1178 (187.175, -31.35) -> (187.175, -32.5)
  arc A414 (186.975, -32.7) -> (187.175, -32.5) centre (186.975, -32.5) ccw
  line L1179 (186.975, -32.7) -> (185.725, -32.7)
  line L1180 (185.725, -32.7) -> (185.725, -33.8)
  line L1181 (185.725, -33.8) -> (186.975, -33.8)
  arc A415 (187.175, -34) -> (186.975, -33.8) centre (186.975, -34) ccw
  line L1182 (201.425, -53) -> (201.425, -54.15)
  line L1183 (201.425, -54.15) -> (202.325, -54.15)
  line L1184 (202.325, -54.15) -> (202.325, -53)
  arc A416 (202.525, -52.8) -> (202.325, -53) centre (202.525, -53) ccw
  line L1185 (202.525, -52.8) -> (203.775, -52.8)
  line L1186 (203.775, -52.8) -> (203.775, -51.7)
  line L1187 (203.775, -51.7) -> (202.525, -51.7)
  arc A417 (202.325, -51.5) -> (202.525, -51.7) centre (202.525, -51.5) ccw
  line L1188 (202.325, -51.5) -> (202.325, -50.35)
  line L1189 (202.325, -50.35) -> (201.425, -50.35)
  line L1190 (201.425, -50.35) -> (201.425, -51.5)
  arc A418 (201.225, -51.7) -> (201.425, -51.5) centre (201.225, -51.5) ccw
  line L1191 (201.225, -51.7) -> (199.975, -51.7)
  line L1192 (199.975, -51.7) -> (199.975, -52.8)
  line L1193 (199.975, -52.8) -> (201.225, -52.8)
  arc A419 (201.425, -53) -> (201.225, -52.8) centre (201.225, -53) ccw
  line L1194 (177.675, -53) -> (177.675, -54.15)
  line L1195 (177.675, -54.15) -> (178.575, -54.15)
  line L1196 (178.575, -54.15) -> (178.575, -53)
  arc A420 (178.775, -52.8) -> (178.575, -53) centre (178.775, -53) ccw
  line L1197 (178.775, -52.8) -> (180.025, -52.8)
  line L1198 (180.025, -52.8) -> (180.025, -51.7)
  line L1199 (180.025, -51.7) -> (178.775, -51.7)
  arc A421 (178.575, -51.5) -> (178.775, -51.7) centre (178.775, -51.5) ccw
  line L1200 (178.575, -51.5) -> (178.575, -50.35)
  line L1201 (178.575, -50.35) -> (177.675, -50.35)
  line L1202 (177.675, -50.35) -> (177.675, -51.5)
  arc A422 (177.475, -51.7) -> (177.675, -51.5) centre (177.475, -51.5) ccw
  line L1203 (177.475, -51.7) -> (176.225, -51.7)
  line L1204 (176.225, -51.7) -> (176.225, -52.8)
  line L1205 (176.225, -52.8) -> (177.475, -52.8)
  arc A423 (177.675, -53) -> (177.475, -52.8) centre (177.475, -53) ccw
  line L1206 (153.925, -53) -> (153.925, -54.15)
  line L1207 (153.925, -54.15) -> (154.825, -54.15)
  line L1208 (154.825, -54.15) -> (154.825, -53)
  arc A424 (155.025, -52.8) -> (154.825, -53) centre (155.025, -53) ccw
  line L1209 (155.025, -52.8) -> (156.275, -52.8)
  line L1210 (156.275, -52.8) -> (156.275, -51.7)
  line L1211 (156.275, -51.7) -> (155.025, -51.7)
  arc A425 (154.825, -51.5) -> (155.025, -51.7) centre (155.025, -51.5) ccw
  line L1212 (154.825, -51.5) -> (154.825, -50.35)
  line L1213 (154.825, -50.35) -> (153.925, -50.35)
  line L1214 (153.925, -50.35) -> (153.925, -51.5)
  arc A426 (153.725, -51.7) -> (153.925, -51.5) centre (153.725, -51.5) ccw
  line L1215 (153.725, -51.7) -> (152.475, -51.7)
  line L1216 (152.475, -51.7) -> (152.475, -52.8)
  line L1217 (152.475, -52.8) -> (153.725, -52.8)
  arc A427 (153.925, -53) -> (153.725, -52.8) centre (153.725, -53) ccw
  line L1218 (70.8, -53) -> (70.8, -54.15)
  line L1219 (70.8, -54.15) -> (71.7, -54.15)
  line L1220 (71.7, -54.15) -> (71.7, -53)
  arc A428 (71.9, -52.8) -> (71.7, -53) centre (71.9, -53) ccw
  line L1221 (71.9, -52.8) -> (73.15, -52.8)
  line L1222 (73.15, -52.8) -> (73.15, -51.7)
  line L1223 (73.15, -51.7) -> (71.9, -51.7)
  arc A429 (71.7, -51.5) -> (71.9, -51.7) centre (71.9, -51.5) ccw
  line L1224 (71.7, -51.5) -> (71.7, -50.35)
  line L1225 (71.7, -50.35) -> (70.8, -50.35)
  line L1226 (70.8, -50.35) -> (70.8, -51.5)
  arc A430 (70.6, -51.7) -> (70.8, -51.5) centre (70.6, -51.5) ccw
  line L1227 (70.6, -51.7) -> (69.35, -51.7)
  line L1228 (69.35, -51.7) -> (69.35, -52.8)
  line L1229 (69.35, -52.8) -> (70.6, -52.8)
  arc A431 (70.8, -53) -> (70.6, -52.8) centre (70.6, -53) ccw
  line L1230 (-68.75, 45.25) -> (-54.75, 45.25)
  line L1231 (-54.75, 45.25) -> (-54.75, 59.25)
  line L1232 (-54.75, 59.25) -> (-68.75, 59.25)
  line L1233 (-68.75, 59.25) -> (-68.75, 45.25)
  line L1234 (-68.75, 45.25) -> (-54.75, 59.25) construction
  line L1235 (-54.75, 45.25) -> (-68.75, 59.25) construction
  line L1236 (-30.75, 45.25) -> (-16.75, 45.25)
  line L1237 (-16.75, 45.25) -> (-16.75, 59.25)
  line L1238 (-16.75, 59.25) -> (-30.75, 59.25)
  line L1239 (-30.75, 59.25) -> (-30.75, 45.25)
  line L1240 (-30.75, 45.25) -> (-16.75, 59.25) construction
  line L1241 (-16.75, 45.25) -> (-30.75, 59.25) construction
  line L1242 (-11.75, 45.25) -> (2.25, 45.25)
  line L1243 (2.25, 45.25) -> (2.25, 59.25)
  line L1244 (2.25, 59.25) -> (-11.75, 59.25)
  line L1245 (-11.75, 59.25) -> (-11.75, 45.25)
  line L1246 (-11.75, 45.25) -> (2.25, 59.25) construction
  line L1247 (2.25, 45.25) -> (-11.75, 59.25) construction
  line L1248 (7.25, 45.25) -> (21.25, 45.25)
  line L1249 (21.25, 45.25) -> (21.25, 59.25)
  line L1250 (21.25, 59.25) -> (7.25, 59.25)
  line L1251 (7.25, 59.25) -> (7.25, 45.25)
  line L1252 (7.25, 45.25) -> (21.25, 59.25) construction
  line L1253 (21.25, 45.25) -> (7.25, 59.25) construction
  line L1254 (26.25, 45.25) -> (40.25, 45.25)
  line L1255 (40.25, 45.25) -> (40.25, 59.25)
  line L1256 (40.25, 59.25) -> (26.25, 59.25)
  line L1257 (26.25, 59.25) -> (26.25, 45.25)
  line L1258 (26.25, 45.25) -> (40.25, 59.25) construction
  line L1259 (40.25, 45.25) -> (26.25, 59.25) construction
  line L1260 (54.75, 45.25) -> (68.75, 45.25)
  line L1261 (68.75, 45.25) -> (68.75, 59.25)
  line L1262 (68.75, 59.25) -> (54.75, 59.25)
  line L1263 (54.75, 59.25) -> (54.75, 45.25)
  line L1264 (54.75, 45.25) -> (68.75, 59.25) construction
  line L1265 (68.75, 45.25) -> (54.75, 59.25) construction
  line L1266 (73.75, 45.25) -> (87.75, 45.25)
  line L1267 (73.75, 59.25) -> (73.75, 45.25)
  line L1268 (87.75, 45.25) -> (87.75, 59.25)
  line L1269 (87.75, 59.25) -> (73.75, 59.25)
  line L1270 (73.75, 45.25) -> (87.75, 59.25) construction
  line L1271 (87.75, 45.25) -> (73.75, 59.25) construction
  line L1272 (92.75, 45.25) -> (106.75, 45.25)
  line L1273 (92.75, 59.25) -> (92.75, 45.25)
  line L1274 (106.75, 45.25) -> (106.75, 59.25)
  line L1275 (106.75, 59.25) -> (92.75, 59.25)
  line L1276 (92.75, 45.25) -> (106.75, 59.25) construction
  line L1277 (106.75, 45.25) -> (92.75, 59.25) construction
  line L1278 (111.75, 45.25) -> (125.75, 45.25)
  line L1279 (111.75, 59.25) -> (111.75, 45.25)
  line L1280 (125.75, 45.25) -> (125.75, 59.25)
  line L1281 (125.75, 59.25) -> (111.75, 59.25)
  line L1282 (111.75, 45.25) -> (125.75, 59.25) construction
  line L1283 (125.75, 45.25) -> (111.75, 59.25) construction
  line L1284 (140.25, 45.25) -> (154.25, 45.25)
  line L1285 (154.25, 45.25) -> (154.25, 59.25)
  line L1286 (154.25, 59.25) -> (140.25, 59.25)
  line L1287 (140.25, 59.25) -> (140.25, 45.25)
  line L1288 (140.25, 45.25) -> (154.25, 59.25) construction
  line L1289 (154.25, 45.25) -> (140.25, 59.25) construction
  line L1290 (173.25, 45.25) -> (173.25, 59.25)
  line L1291 (159.25, 45.25) -> (173.25, 45.25)
  line L1292 (159.25, 59.25) -> (159.25, 45.25)
  line L1293 (173.25, 59.25) -> (159.25, 59.25)
  line L1294 (173.25, 45.25) -> (159.25, 59.25) construction
  line L1295 (159.25, 45.25) -> (173.25, 59.25) construction
  line L1296 (192.25, 45.25) -> (192.25, 59.25)
  line L1297 (178.25, 45.25) -> (192.25, 45.25)
  line L1298 (178.25, 59.25) -> (178.25, 45.25)
  line L1299 (192.25, 59.25) -> (178.25, 59.25)
  line L1300 (192.25, 45.25) -> (178.25, 59.25) construction
  line L1301 (178.25, 45.25) -> (192.25, 59.25) construction
  line L1302 (211.25, 45.25) -> (211.25, 59.25)
  line L1303 (197.25, 45.25) -> (211.25, 45.25)
  line L1304 (197.25, 59.25) -> (197.25, 45.25)
  line L1305 (211.25, 59.25) -> (197.25, 59.25)
  line L1306 (211.25, 45.25) -> (197.25, 59.25) construction
  line L1307 (197.25, 45.25) -> (211.25, 59.25) construction
  line L1308 (-211.25, 16.75) -> (-197.25, 16.75)
  line L1309 (-197.25, 16.75) -> (-197.25, 30.75)
  line L1310 (-197.25, 30.75) -> (-211.25, 30.75)
  line L1311 (-211.25, 30.75) -> (-211.25, 16.75)
  line L1312 (-211.25, 16.75) -> (-197.25, 30.75) construction
  line L1313 (-197.25, 16.75) -> (-211.25, 30.75) construction
  line L1314 (-178.25, 30.75) -> (-192.25, 30.75)
  line L1315 (-178.25, 16.75) -> (-178.25, 30.75)
  line L1316 (-192.25, 30.75) -> (-192.25, 16.75)
  line L1317 (-192.25, 16.75) -> (-178.25, 16.75)
  line L1318 (-192.25, 16.75) -> (-178.25, 30.75) construction
  line L1319 (-178.25, 16.75) -> (-192.25, 30.75) construction
  line L1320 (-159.25, 30.75) -> (-173.25, 30.75)
  line L1321 (-159.25, 16.75) -> (-159.25, 30.75)
  line L1322 (-173.25, 30.75) -> (-173.25, 16.75)
  line L1323 (-173.25, 16.75) -> (-159.25, 16.75)
  line L1324 (-173.25, 16.75) -> (-159.25, 30.75) construction
  line L1325 (-159.25, 16.75) -> (-173.25, 30.75) construction
  line L1326 (-197.25, 11.75) -> (-211.25, 11.75)
  line L1327 (-197.25, -2.25) -> (-197.25, 11.75)
  line L1328 (-211.25, 11.75) -> (-211.25, -2.25)
  line L1329 (-211.25, -2.25) -> (-197.25, -2.25)
  line L1330 (-211.25, -2.25) -> (-197.25, 11.75) construction
  line L1331 (-197.25, -2.25) -> (-211.25, 11.75) construction
  line L1332 (-178.25, 11.75) -> (-192.25, 11.75)
  line L1333 (-178.25, -2.25) -> (-178.25, 11.75)
  line L1334 (-192.25, 11.75) -> (-192.25, -2.25)
  line L1335 (-192.25, -2.25) -> (-178.25, -2.25)
  line L1336 (-192.25, -2.25) -> (-178.25, 11.75) construction
  line L1337 (-178.25, -2.25) -> (-192.25, 11.75) construction
  line L1338 (-159.25, 11.75) -> (-173.25, 11.75)
  line L1339 (-159.25, -2.25) -> (-159.25, 11.75)
  line L1340 (-173.25, 11.75) -> (-173.25, -2.25)
  line L1341 (-173.25, -2.25) -> (-159.25, -2.25)
  line L1342 (-173.25, -2.25) -> (-159.25, 11.75) construction
  line L1343 (-159.25, -2.25) -> (-173.25, 11.75) construction
  line L1344 (-197.25, -7.25) -> (-211.25, -7.25)
  line L1345 (-197.25, -21.25) -> (-197.25, -7.25)
  line L1346 (-211.25, -7.25) -> (-211.25, -21.25)
  line L1347 (-211.25, -21.25) -> (-197.25, -21.25)
  line L1348 (-211.25, -21.25) -> (-197.25, -7.25) construction
  line L1349 (-197.25, -21.25) -> (-211.25, -7.25) construction
  line L1350 (-178.25, -7.25) -> (-192.25, -7.25)
  line L1351 (-178.25, -21.25) -> (-178.25, -7.25)
  line L1352 (-192.25, -7.25) -> (-192.25, -21.25)
  line L1353 (-192.25, -21.25) -> (-178.25, -21.25)
  line L1354 (-192.25, -21.25) -> (-178.25, -7.25) construction
  line L1355 (-178.25, -21.25) -> (-192.25, -7.25) construction
  line L1356 (-159.25, -7.25) -> (-173.25, -7.25)
  line L1357 (-159.25, -21.25) -> (-159.25, -7.25)
  line L1358 (-173.25, -7.25) -> (-173.25, -21.25)
  line L1359 (-173.25, -21.25) -> (-159.25, -21.25)
  line L1360 (-173.25, -21.25) -> (-159.25, -7.25) construction
  line L1361 (-159.25, -21.25) -> (-173.25, -7.25) construction
  line L1362 (-197.25, -26.25) -> (-211.25, -26.25)
  line L1363 (-197.25, -40.25) -> (-197.25, -26.25)
  line L1364 (-211.25, -26.25) -> (-211.25, -40.25)
  line L1365 (-211.25, -40.25) -> (-197.25, -40.25)
  line L1366 (-211.25, -40.25) -> (-197.25, -26.25) construction
  line L1367 (-197.25, -40.25) -> (-211.25, -26.25) construction
  line L1368 (-178.25, -26.25) -> (-192.25, -26.25)
  line L1369 (-178.25, -40.25) -> (-178.25, -26.25)
  line L1370 (-192.25, -26.25) -> (-192.25, -40.25)
  line L1371 (-192.25, -40.25) -> (-178.25, -40.25)
  line L1372 (-192.25, -40.25) -> (-178.25, -26.25) construction
  line L1373 (-178.25, -40.25) -> (-192.25, -26.25) construction
  line L1374 (-159.25, -26.25) -> (-173.25, -26.25)
  line L1375 (-159.25, -40.25) -> (-159.25, -26.25)
  line L1376 (-173.25, -26.25) -> (-173.25, -40.25)
  line L1377 (-173.25, -40.25) -> (-159.25, -40.25)
  line L1378 (-173.25, -40.25) -> (-159.25, -26.25) construction
  line L1379 (-159.25, -40.25) -> (-173.25, -26.25) construction
  line L1380 (-197.25, -45.25) -> (-211.25, -45.25)
  line L1381 (-197.25, -59.25) -> (-197.25, -45.25)
  line L1382 (-211.25, -45.25) -> (-211.25, -59.25)
  line L1383 (-211.25, -59.25) -> (-197.25, -59.25)
  line L1384 (-211.25, -59.25) -> (-197.25, -45.25) construction
  line L1385 (-197.25, -59.25) -> (-211.25, -45.25) construction
  line L1386 (-178.25, -45.25) -> (-192.25, -45.25)
  line L1387 (-178.25, -59.25) -> (-178.25, -45.25)
  line L1388 (-192.25, -45.25) -> (-192.25, -59.25)
  line L1389 (-192.25, -59.25) -> (-178.25, -59.25)
  line L1390 (-192.25, -59.25) -> (-178.25, -45.25) construction
  line L1391 (-178.25, -59.25) -> (-192.25, -45.25) construction
  line L1392 (-159.25, -45.25) -> (-173.25, -45.25)
  line L1393 (-159.25, -59.25) -> (-159.25, -45.25)
  line L1394 (-173.25, -45.25) -> (-173.25, -59.25)
  line L1395 (-173.25, -59.25) -> (-159.25, -59.25)
  line L1396 (-173.25, -59.25) -> (-159.25, -45.25) construction
  line L1397 (-159.25, -59.25) -> (-173.25, -45.25) construction
  line L1398 (-154.25, 16.75) -> (-140.25, 16.75)
  line L1399 (-140.25, 16.75) -> (-140.25, 30.75)
  line L1400 (-140.25, 30.75) -> (-154.25, 30.75)
  line L1401 (-154.25, 30.75) -> (-154.25, 16.75)
  line L1402 (-154.25, 16.75) -> (-140.25, 30.75) construction
  line L1403 (-140.25, 16.75) -> (-154.25, 30.75) construction
  line L1404 (-154.25, -11.75) -> (-140.25, -11.75)
  line L1405 (-140.25, -11.75) -> (-140.25, 2.25)
  line L1406 (-140.25, 2.25) -> (-154.25, 2.25)
  line L1407 (-154.25, 2.25) -> (-154.25, -11.75)
  line L1408 (-154.25, -11.75) -> (-140.25, 2.25) construction
  line L1409 (-140.25, -11.75) -> (-154.25, 2.25) construction
  line L1410 (-154.25, -49.75) -> (-140.25, -49.75)
  line L1411 (-140.25, -49.75) -> (-140.25, -35.75)
  line L1412 (-140.25, -35.75) -> (-154.25, -35.75)
  line L1413 (-154.25, -35.75) -> (-154.25, -49.75)
  line L1414 (-154.25, -49.75) -> (-140.25, -35.75) construction
  line L1415 (-140.25, -49.75) -> (-154.25, -35.75) construction
  line L1416 (-130.5, -59.25) -> (-116.5, -59.25)
  line L1417 (-116.5, -59.25) -> (-116.5, -45.25)
  line L1418 (-116.5, -45.25) -> (-130.5, -45.25)
  line L1419 (-130.5, -45.25) -> (-130.5, -59.25)
  line L1420 (-130.5, -59.25) -> (-116.5, -45.25) construction
  line L1421 (-116.5, -59.25) -> (-130.5, -45.25) construction
  line L1422 (-111.5, -59.25) -> (-97.5, -59.25)
  line L1423 (-97.5, -59.25) -> (-97.5, -45.25)
  line L1424 (-97.5, -45.25) -> (-111.5, -45.25)
  line L1425 (-111.5, -45.25) -> (-111.5, -59.25)
  line L1426 (-111.5, -59.25) -> (-97.5, -45.25) construction
  line L1427 (-97.5, -59.25) -> (-111.5, -45.25) construction
  line L1428 (-92.5, -59.25) -> (-78.5, -59.25)
  line L1429 (-78.5, -59.25) -> (-78.5, -45.25)
  line L1430 (-78.5, -45.25) -> (-92.5, -45.25)
  line L1431 (-92.5, -45.25) -> (-92.5, -59.25)
  line L1432 (-92.5, -59.25) -> (-78.5, -45.25) construction
  line L1433 (-78.5, -59.25) -> (-92.5, -45.25) construction
  line L1434 (-97.5, -40.25) -> (-111.5, -40.25)
  line L1435 (-111.5, -40.25) -> (-111.5, -26.25)
  line L1436 (-111.5, -26.25) -> (-97.5, -26.25)
  line L1437 (-97.5, -26.25) -> (-97.5, -40.25)
  line L1438 (-97.5, -40.25) -> (-111.5, -26.25) construction
  line L1439 (-111.5, -40.25) -> (-97.5, -26.25) construction
  line L1440 (-130.5, 16.75) -> (-116.5, 16.75)
  line L1441 (-116.5, 16.75) -> (-116.5, 30.75)
  line L1442 (-116.5, 30.75) -> (-130.5, 30.75)
  line L1443 (-130.5, 30.75) -> (-130.5, 16.75)
  line L1444 (-130.5, 16.75) -> (-116.5, 30.75) construction
  line L1445 (-116.5, 16.75) -> (-130.5, 30.75) construction
  line L1446 (-97.5, 30.75) -> (-111.5, 30.75)
  line L1447 (-97.5, 16.75) -> (-97.5, 30.75)
  line L1448 (-111.5, 30.75) -> (-111.5, 16.75)
  line L1449 (-111.5, 16.75) -> (-97.5, 16.75)
  line L1450 (-97.5, 16.75) -> (-111.5, 30.75) construction
  line L1451 (-111.5, 16.75) -> (-97.5, 30.75) construction
  line L1452 (-78.5, 30.75) -> (-92.5, 30.75)
  line L1453 (-78.5, 16.75) -> (-78.5, 30.75)
  line L1454 (-92.5, 30.75) -> (-92.5, 16.75)
  line L1455 (-92.5, 16.75) -> (-78.5, 16.75)
  line L1456 (-78.5, 16.75) -> (-92.5, 30.75) construction
  line L1457 (-92.5, 16.75) -> (-78.5, 30.75) construction
  line L1458 (-116.5, 11.75) -> (-130.5, 11.75)
  line L1459 (-116.5, -2.25) -> (-116.5, 11.75)
  line L1460 (-130.5, 11.75) -> (-130.5, -2.25)
  line L1461 (-130.5, -2.25) -> (-116.5, -2.25)
  line L1462 (-116.5, -2.25) -> (-130.5, 11.75) construction
  line L1463 (-130.5, -2.25) -> (-116.5, 11.75) construction
  line L1464 (-97.5, 11.75) -> (-111.5, 11.75)
  line L1465 (-97.5, -2.25) -> (-97.5, 11.75)
  line L1466 (-111.5, 11.75) -> (-111.5, -2.25)
  line L1467 (-111.5, -2.25) -> (-97.5, -2.25)
  line L1468 (-97.5, -2.25) -> (-111.5, 11.75) construction
  line L1469 (-111.5, -2.25) -> (-97.5, 11.75) construction
  line L1470 (-78.5, 11.75) -> (-92.5, 11.75)
  line L1471 (-78.5, -2.25) -> (-78.5, 11.75)
  line L1472 (-92.5, 11.75) -> (-92.5, -2.25)
  line L1473 (-92.5, -2.25) -> (-78.5, -2.25)
  line L1474 (-78.5, -2.25) -> (-92.5, 11.75) construction
  line L1475 (-92.5, -2.25) -> (-78.5, 11.75) construction
  line L1476 (-68.75, 16.75) -> (-54.75, 16.75)
  line L1477 (-54.75, 16.75) -> (-54.75, 30.75)
  line L1478 (-54.75, 30.75) -> (-68.75, 30.75)
  line L1479 (-68.75, 30.75) -> (-68.75, 16.75)
  line L1480 (-68.75, 16.75) -> (-54.75, 30.75) construction
  line L1481 (-54.75, 16.75) -> (-68.75, 30.75) construction
  line L1482 (-35.75, 16.75) -> (-35.75, 30.75)
  line L1483 (-49.75, 30.75) -> (-49.75, 16.75)
  line L1484 (-35.75, 30.75) -> (-49.75, 30.75)
  line L1485 (-49.75, 16.75) -> (-35.75, 16.75)
  line L1486 (-49.75, 16.75) -> (-35.75, 30.75) construction
  line L1487 (-35.75, 16.75) -> (-49.75, 30.75) construction
  line L1488 (-16.75, 16.75) -> (-16.75, 30.75)
  line L1489 (-30.75, 30.75) -> (-30.75, 16.75)
  line L1490 (-16.75, 30.75) -> (-30.75, 30.75)
  line L1491 (-30.75, 16.75) -> (-16.75, 16.75)
  line L1492 (-30.75, 16.75) -> (-16.75, 30.75) construction
  line L1493 (-16.75, 16.75) -> (-30.75, 30.75) construction
  line L1494 (2.25, 16.75) -> (2.25, 30.75)
  line L1495 (-11.75, 30.75) -> (-11.75, 16.75)
  line L1496 (2.25, 30.75) -> (-11.75, 30.75)
  line L1497 (-11.75, 16.75) -> (2.25, 16.75)
  line L1498 (-11.75, 16.75) -> (2.25, 30.75) construction
  line L1499 (2.25, 16.75) -> (-11.75, 30.75) construction
  line L1500 (21.25, 16.75) -> (21.25, 30.75)
  line L1501 (7.25, 30.75) -> (7.25, 16.75)
  line L1502 (21.25, 30.75) -> (7.25, 30.75)
  line L1503 (7.25, 16.75) -> (21.25, 16.75)
  line L1504 (7.25, 16.75) -> (21.25, 30.75) construction
  line L1505 (21.25, 16.75) -> (7.25, 30.75) construction
  line L1506 (40.25, 16.75) -> (40.25, 30.75)
  line L1507 (26.25, 30.75) -> (26.25, 16.75)
  line L1508 (40.25, 30.75) -> (26.25, 30.75)
  line L1509 (26.25, 16.75) -> (40.25, 16.75)
  line L1510 (26.25, 16.75) -> (40.25, 30.75) construction
  line L1511 (40.25, 16.75) -> (26.25, 30.75) construction
  line L1512 (59.25, 16.75) -> (59.25, 30.75)
  line L1513 (45.25, 30.75) -> (45.25, 16.75)
  line L1514 (59.25, 30.75) -> (45.25, 30.75)
  line L1515 (45.25, 16.75) -> (59.25, 16.75)
  line L1516 (45.25, 16.75) -> (59.25, 30.75) construction